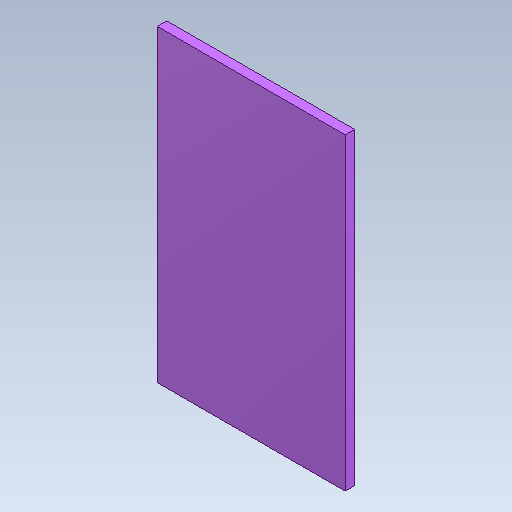
# Autodesk Inventor part: 2717_1.000000
Saved by Autodesk Inventor 2020 (Build 240168000, 168)
## iProperties
Created: 2019-07-14
Part Number: 2717_1.000000
Material: Generic
Document SubType Name: Modeling
Designer: psrob
Density: 1 g/cm^3
Appearance: 2717_1.000000, 2717_1.000000
Author: psrob
Autodesk Inventor part; units mm, degrees
ref_plane "YZ Plane" through (0, 0, 0) normal (1, 0, 0) x (0, 1, 0)
ref_plane "XZ Plane" through (0, 0, 0) normal (0, 1, 0) x (-1, 0, 0)
ref_plane "XY Plane" through (0, 0, 0) normal (0, 0, 1) x (1, 0, 0)
sketch "2717_1.000000, 2717_1.000000_20" plane through (0, 0, 0) normal (0, 0, 1) x (1, 0, 0)
  line L0 (-9.89, 16.24) -> (9.89, 16.24)
  line L1 (9.89, 16.24) -> (9.89, -16.24)
  line L2 (9.89, -16.24) -> (-9.89, -16.24)
  line L3 (-9.89, -16.24) -> (-9.89, 16.24)
  constraints: 8 end point
extrude "Extrusion1" add sketch "2717_1.000000, 2717_1.000000_20" along normal blind 1
body "Solid1"
